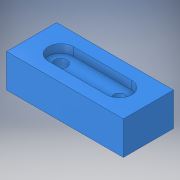
# Autodesk Inventor part: AirPressureAndValvePart2
Saved by Autodesk Inventor 2018 (Build 220112000, 112)
## iProperties
Created: 2020-03-27
Part Number: AirPressureAndValvePart2
Material: Generic
Document SubType Name: Modeling
Designer: emile
Density: 1 g/cm^3
Appearance: Cyan
Author: emile
Autodesk Inventor part; units mm, degrees
ref_plane "YZ Plane" through (0, 0, 0) normal (1, 0, 0) x (0, 1, 0)
ref_plane "XZ Plane" through (0, 0, 0) normal (0, 1, 0) x (-1, 0, 0)
ref_plane "XY Plane" through (0, 0, 0) normal (0, 0, 1) x (1, 0, 0)
sketch "Sketch1" plane through (0, 0, 0) normal (0, 1, 0) x (-1, 0, 0)
  line L0 (-44.45, -19.05) -> (44.45, -19.05)
  line L1 (44.45, -19.05) -> (44.45, 19.05)
  line L2 (44.45, 19.05) -> (-44.45, 19.05)
  line L3 (-44.45, 19.05) -> (-44.45, -19.05)
  line L4 (-44.45, -19.05) -> (44.45, 19.05) construction
  line L5 (44.45, -19.05) -> (-44.45, 19.05) construction
  circle A0 centre (22.225, 0) radius 3.9688
  circle A1 centre (-22.225, 0) radius 3.9688
  circle A2 centre (22.225, 0) radius 12.7
  circle A3 centre (-22.225, 0) radius 12.7
  point P0 (0, 0)
  point P1 (0, 0)
  point P2 (0, 0)
  dimension "d3" = 38.1
  dimension "d4" = 88.9
  dimension "d20" = 7.9375
  dimension "d21" = 25.4
  dimension "d22" = 22.225
  dimension "d23" = 22.225
  constraints: 12 end point, 4 centre point, 4 midpoint, 2 coincident, 2 equal radius, 2 horizontal alignment, 2 parallel, 1 horizontal, 1 perpendicular
  measures "d3" distance of L0.end L1.end
  measures "d4" distance of L0.start L0.end
  measures "d20" diameter of A0
  measures "d21" diameter of A2
  measures "d22" distance of point (0, 0) A2.centre
  measures "d23" distance of point (0, 0) A3.centre
extrude "Extrusion5" add sketch "Sketch1" along normal blind 25.4 contours L3 L2 L1 L0 | A2 | A3
sketch "Sketch10" plane through (0, 25.4, 0) normal (0, 1, 0) x (1, 0, 0)
  circle A0 centre (22.225, 0) radius 3.9687 projected
  circle A1 centre (-22.225, 0) radius 3.9687 projected
  line L0 (44.45, 19.05) -> (-44.45, 19.05) projected
  line L1 (-44.45, 19.05) -> (-44.45, -19.05) projected
  line L2 (-44.45, -19.05) -> (44.45, -19.05) projected
  line L3 (44.45, -19.05) -> (44.45, 19.05) projected
  circle A2 centre (-22.225, 0) radius 4.826
  circle A3 centre (-22.225, 0) radius 9.525
  point P0 (0, 0)
  dimension "d38" = 9.652
  dimension "d41" = 19.05
  constraints: 2 centre point, 2 coincident
  measures "d38" diameter of A2
  measures "d41" diameter of A3
extrude "Extrusion8" cut sketch "Sketch10" against normal blind 19.05 contours A2
extrude "Extrusion9" cut sketch "Sketch10" against normal blind 6.35 contours A3
sketch "Sketch12" plane through (0, 25.4, 0) normal (0, 1, 0) x (1, 0, 0)
  circle A0 centre (-22.225, 0) radius 9.525 projected
  circle A1 centre (22.225, 0) radius 3.9687 projected
  line L0 (44.45, 19.05) -> (-44.45, 19.05) projected
  line L1 (-44.45, 19.05) -> (-44.45, -19.05) projected
  line L2 (-44.45, -19.05) -> (44.45, -19.05) projected
  line L3 (44.45, -19.05) -> (44.45, 19.05) projected
  circle A2 centre (-22.225, 0) radius 3.9687 projected
  line L4 (-22.225, 0) -> (22.225, 0) construction
  line L5 (-22.225, -9.525) -> (22.225, -9.525)
  line L6 (22.225, 9.525) -> (-22.225, 9.525)
  arc A3 (-22.225, 9.525) -> (-22.225, -9.525) centre (-22.225, 0) ccw
  arc A4 (22.225, -9.525) -> (22.225, 9.525) centre (22.225, 0) ccw
  point P0 (0, 0)
  point P1 (0, 0)
  constraints: 8 end point, 5 tangent, 4 point on circle, 2 centre point, 1 horizontal, 1 midpoint, 1 parallel
extrude "Extrusion10" cut sketch "Sketch12" against normal up to surface (6.35 mm away) contours A0 | A0 L6 A4 L5
equation "\"d23\" = d22"
body "Solid2"
